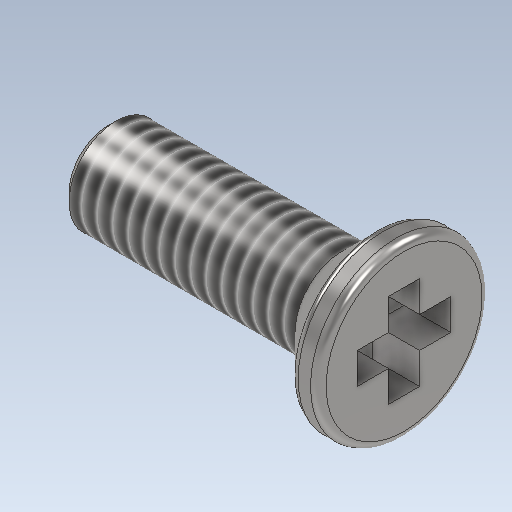
# Autodesk Inventor part: M3_Short_Bolt
Saved by Autodesk Inventor 2021 (Build 250183000, 183)
## iProperties
Created: 2020-01-05
Part Number: M3_Short_Bolt
Material: Steel, Alloy
Document SubType Name: Modeling
Designer: ermoz
Density: 7.73 g/cm^3
Appearance: Semi-Polished
Mass: 0.626508 g
Surface Area: 1.52538 cm^2
Volume: 0.0810489 cm^3
Author: ermoz
Autodesk Inventor part; units mm, degrees
ref_plane "YZ Plane" through (0, 0, 0) normal (1, 0, 0) x (0, 1, 0)
ref_plane "XZ Plane" through (0, 0, 0) normal (0, 1, 0) x (-1, 0, 0)
ref_plane "XY Plane" through (0, 0, 0) normal (0, 0, 1) x (1, 0, 0)
sketch "Sketch1" plane through (0, 0, 0) normal (0, 1, 0) x (-1, 0, 0)
  line L0 (0, 0) -> (0, -2.75)
  line L1 (0, 0) -> (9.5, 0)
  line L2 (9.5, 0) -> (9.5, -1.5)
  line L3 (9.5, -1.5) -> (2, -1.5)
  line L4 (2, -1.5) -> (0.75, -2.75)
  line L5 (2, -1.5) -> (3.7678, -1.5) construction
  line L6 (0.75, -2.75) -> (0, -2.75)
  dimension "d0" = 2.75
  dimension "d1" = 9.5
  dimension "d2" = 1.5
  dimension "d3" = 7.5
  dimension "d4" = 135
  constraints: 14 end point, 4 horizontal, 2 vertical, 1 equal length
  measures "d0" distance of L0.start L0.end
  measures "d1" distance of L0.start L1.end
  measures "d2" distance of L1.end L2.end
  measures "d3" distance of L2.end L3.end
  measures "d4" angle of L4 L5
revolve "Revolution1" add sketch "Sketch1" angle 360 about axis through (0, 0, 0) along (-1, 0, 0)
thread "Thread1" size "M3x0.5" class "6g" standard "ANSI Metric M Profile" full length
fillet "Fillet1" radius 0.25 2 edges at (-0.75, 0, 2.75) (0, 0, 2.75)
sketch "Sketch2" plane through (0, 0, 0) normal (1, 0, 0) x (0, 0, -1)
  line L0 (-1.5, 0.5) -> (1.5, 0.5)
  line L1 (1.5, 0.5) -> (1.5, -0.5)
  line L2 (1.5, -0.5) -> (-1.5, -0.5)
  line L3 (-1.5, -0.5) -> (-1.5, 0.5)
  line L4 (-1.5, 0.5) -> (1.5, -0.5) construction
  line L5 (1.5, 0.5) -> (-1.5, -0.5) construction
  line L6 (0.5, 1.5) -> (-0.5, 1.5)
  line L7 (-0.5, 1.5) -> (-0.5, -1.5)
  line L8 (-0.5, -1.5) -> (0.5, -1.5)
  line L9 (0.5, -1.5) -> (0.5, 1.5)
  line L10 (0.5, 1.5) -> (-0.5, -1.5) construction
  line L11 (-0.5, 1.5) -> (0.5, -1.5) construction
  point P0 (0, 0)
  point P1 (0.5, 0.5)
  point P2 (-0.5, 0.5)
  point P3 (-0.5, -0.5)
  point P4 (0.5, -0.5)
  dimension "d9" = 3
  dimension "d10" = 1
  dimension "d11" = 1
  dimension "d12" = 3
  constraints: 24 end point, 4 midpoint, 4 parallel, 2 horizontal, 2 perpendicular
  measures "d9" distance of L1.end L2.end
  measures "d10" distance of L0.end L1.end
  measures "d11" distance of L8.end L7.end
  measures "d12" distance of L7.end L6.end
extrude "Extrusion1" cut sketch "Sketch2" against normal blind 1.5
chamfer "Chamfer1" distance 0.25 angle 45 1 edges at (-9.5, 0, 1.5)
body "Solid1"
